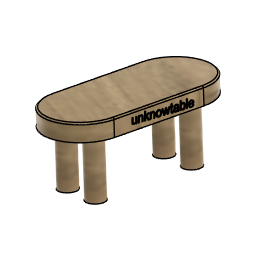
day 5 table (Autodesk Fusion 360 design; units mm, degrees)
Autodesk Fusion 360 part; units mm, degrees
sketch "Sketch1" plane through (0, 0, 0) normal (0, 0, 1) x (1, 0, 0)
  line L0 (-30.5248, -10.3271) -> (20.8396, -31.9068)
  arc A0 (20.8396, -31.9068) -> (38.0932, 9.1604) centre (29.4664, -11.3732) ccw
  line L1 (38.0932, 9.1604) -> (-13.2713, 30.7401)
  arc A1 (-13.2713, 30.7401) -> (-30.5248, -10.3271) centre (-21.8981, 10.2065) ccw
  line L2 (-42.4317, 18.8333) -> (50, -20) construction
  constraint tangent L0 A0
  constraint tangent A0 L1
  constraint parallel L0 L1
  constraint tangent L1 A1
  constraint tangent L0 A1
  constraint midpoint A1 L2.start
  constraint midpoint A0 L2.end
extrude "Extrude1" add sketch "Sketch1" along normal blind 10
sketch "Sketch2" plane through (0, 0, 10) normal (0, 0, 1) x (-1, 0, 0)
  arc A0 (13.2713, -30.7401) -> (30.5248, 10.3271) centre (21.8981, -10.2065) ccw
  line L0 (30.5248, 10.3271) -> (-20.8396, 31.9068)
  arc A1 (-20.8396, 31.9068) -> (-38.0932, -9.1604) centre (-29.4664, 11.3732) ccw
  line L1 (-38.0932, -9.1604) -> (13.2713, -30.7401)
  circle A2 centre (19.931, -18.8333) radius 5.4774
extrude "Extrude2" add sketch "Sketch2" along normal blind 35 contours A2
pattern_linear "R-Pattern1" count 2 spacing 60 along (0.921939, -0.387334, 0) count 2 spacing 20 along (-0.387334, -0.921939, 0) of "Extrude2"
move_body "Move1" bodies 1 to x (0.836516, 0.527099, -0.14969) y (0.547668, -0.812937, 0.197972) z (-0.017338, -0.247587, -0.968711) at (-4.4162, 9.3085, 24.5047)
move_body "Move2" bodies 1 to x (0.853719, 0.509637, 0.106932) y (-0.515395, 0.856289, 0.033725) z (-0.074378, -0.083904, 0.993694) at (8.7286, 11.9019, 23.6137)
fillet "Fillet1" radius 0.9 4 edges at (21.361, 17.964, 51.8364) (-4.4904, -30.3742, 53.8588) (-22.2685, 20.4114, 43.1947) (3.5829, 68.7495, 41.1722)
sketch "Sketch3" plane through (29.3756, -1.6479, 5.8184) normal (0.979461, -0.054944, 0.194001) x (0.056009, 0.99843, 0)
  line L0 (46.6401, 42.4234) -> (-8.608, 49.61)
  line L1 (-8.608, 49.61) -> (-9.7818, 40.586)
  line L2 (-9.7818, 40.586) -> (45.4663, 33.3995)
  line L3 (45.4663, 33.3995) -> (46.6401, 42.4234)
  line L4 (1.5781, 42.0477) -> (15.7991, 39.5401) construction
  line L5 (15.7991, 39.5401) -> (16.713, 44.7229) construction
  line L6 (16.713, 44.7229) -> (2.492, 47.2305) construction
  line L7 (2.492, 47.2305) -> (1.5781, 42.0477) construction
  dimension "d11" = 5
  text T0 "unknowtable" font "Arial" height 5 align left top in box 14.4404 x 5.2628 at (1.5781, 42.0477) x (0.984808, -0.173648) y (0.173648, 0.984808) spacing 1
extrude "Extrude3" cut sketch "Sketch3" against normal blind 0.5 text T0
